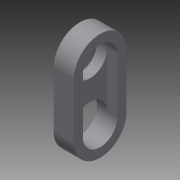
# Autodesk Inventor part: Sensor support
Saved by Autodesk Inventor 2015 (Build 190159000, 159)
## iProperties
Created: 2016-06-05
Part Number: Sensor support
Material: Generic
Document SubType Name: Modeling
Designer: EriveltonDell
Density: 1 g/cm^3
Appearance: Default
Author: EriveltonDell
Autodesk Inventor part; units mm, degrees
ref_plane "YZ Plane" through (0, 0, 0) normal (1, 0, 0) x (0, 1, 0)
ref_plane "XZ Plane" through (0, 0, 0) normal (0, 1, 0) x (-1, 0, 0)
ref_plane "XY Plane" through (0, 0, 0) normal (0, 0, 1) x (1, 0, 0)
sketch "Sketch1" plane through (0, 0, 0) normal (1, 0, 0) x (0, 1, 0)
  arc A0 (18.5, 35) -> (1.5, 35) centre (10, 35) ccw
  arc A1 (1.5, 8) -> (18.5, 8) centre (10, 8) ccw
  arc A2 (23, 35) -> (-3, 35) centre (10, 35) ccw
  arc A3 (-3, 8) -> (23, 8) centre (10, 8) ccw
  line L0 (-3, 35) -> (-3, 8)
  line L1 (23, 35) -> (23, 8)
  circle A4 centre (10, 35) radius 8.5
  circle A5 centre (10, 8) radius 8.5
  dimension "d12" = 17
  dimension "d13" = 17
  dimension "d15" = 26
  dimension "d16" = 26
  constraints: 8 point on circle, 5 centre point, 4 end point, 2 coincident, 1 concentric, 1 horizontal alignment, 1 tangent, 2 other
  measures "d12" diameter of A0
  measures "d13" diameter of A1
  measures "d15" diameter of A2
  measures "d16" diameter of A3
extrude "Extrusion1" add sketch "Sketch1" along normal blind 10
sketch "Sketch2" plane through (10, 0, 0) normal (1, 0, 0) x (0, 0, -1)
  circle A0 centre (-35, 10) radius 8.5
  circle A1 centre (-8, 10) radius 8.5
  circle A2 centre (-8, 10) radius 8.5
  line L0 (-35, 10) -> (-35, 18.5)
  circle A3 centre (-35, 10) radius 8.5
  line L1 (-35, 10) -> (-26.5, 10) construction
  line L2 (-35, 18.5) -> (-7.677334, 18.493873)
  line L3 (-8, 10) -> (-8, 1.5)
  line L4 (-8, 10) -> (0.5, 10) construction
  line L5 (-8, 1.5) -> (-35.117933, 1.500818)
  point P0 (0, 0)
  dimension "d19" = 90
  dimension "d20" = 90
  constraints: 12 end point, 4 point on circle, 2 horizontal, 2 perpendicular, 1 centre point, 1 coincident, 5 other
  measures "d19" angle of L1 L0
  measures "d20" angle of L3 L4
sketch "Sketch2 outline for Extrusion2" plane through (10, 0, 0) normal (1, 0, 0) x (0, 0, -1)
  arc A0 (-8, 1.5) -> (-7.677334, 18.493873) centre (-8, 10) ccw
  line L0 (-35.117933, 1.500818) -> (-8, 1.5)
  arc A1 (-35, 18.5) -> (-35.117933, 1.500818) centre (-35, 10) ccw
  line L1 (-7.677334, 18.493873) -> (-35, 18.5)
extrude "Extrusion2" cut sketch "Sketch2 outline for Extrusion2" against normal blind 5
body "Solid1"
